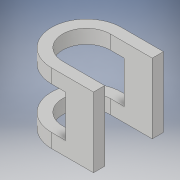
# Autodesk Inventor part: 410571040示範三
Saved by Autodesk Inventor 2017 (Build 210142000, 142)
## iProperties
Part Number: 410571040示範三
Material: 一般
Document SubType Name: Modeling
Designer: user
Density: 1 g/cm^3
Appearance: 預設
Author: user
Autodesk Inventor part; units mm, degrees
ref_plane "YZ Plane" through (0, 0, 0) normal (1, 0, 0) x (0, 1, 0)
ref_plane "XZ Plane" through (0, 0, 0) normal (0, 1, 0) x (-1, 0, 0)
ref_plane "XY Plane" through (0, 0, 0) normal (0, 0, 1) x (1, 0, 0)
sketch "草圖1" plane through (0, 0, 0) normal (0, 1, 0) x (-1, 0, 0)
  line L0 (0, 0) -> (-8, 0)
  line L1 (-8, 0) -> (-8, -30)
  line L2 (0, 0) -> (0, -30)
  arc A0 (-42, -30) -> (-8, -30) centre (-25, -30) ccw
  arc A1 (-50, -30) -> (0, -30) centre (-25, -30) ccw
  line L3 (6.1696, -30) -> (-69.0697, -30) construction
  line L4 (-25, -30) -> (-25, -20.8656)
  line L5 (-42, 0) -> (-42, -30)
  line L6 (-50, 0) -> (-50, -30)
  line L7 (-42, 0) -> (-50, 0)
  dimension "d8" = 30
  dimension "d9" = 8
  dimension "d10" = 25
  dimension "d11" = 17
  constraints: 16 end point, 4 point on circle, 4 point on line, 2 centre point, 2 horizontal, 2 perpendicular, 2 symmetric about line, 2 vertical, 1 coincident
  measures "d8" distance of L0.start L2.end
  measures "d9" distance of L0.start L0.end
  measures "d10" radius of A1
  measures "d11" radius of A0
extrude "擠出1" add sketch "草圖1" along normal blind 10
sketch "草圖2" plane through (0, 10, 0) normal (0, 1, 0) x (1, 0, 0)
  line L0 (0, 30) -> (0, 0) projected
  line L1 (0, 0) -> (0, 20)
  line L2 (0, 20) -> (8, 20)
  line L3 (8, 0) -> (8, 30) projected
  line L4 (8, 20) -> (8, 0)
  line L5 (8, 0) -> (0, 0)
  arc A0 (42, 30) -> (8, 30) centre (25, 30) ccw projected
  line L6 (25, 30) -> (25, 60.7006)
  line L7 (50, 20) -> (50, 0)
  line L8 (50, 0) -> (50, 20)
  line L9 (50, 20) -> (42, 20)
  line L10 (42, 0) -> (42, 20)
  line L11 (42, 20) -> (42, 0)
  line L12 (42, 0) -> (50, 0)
  point P0 (50, 30)
  dimension "d14" = 20
  constraints: 22 end point, 5 symmetric about line, 2 point on line, 2 vertical, 1 horizontal, 1 perpendicular
  measures "d14" distance of L12.start L10.end
extrude "擠出2" add sketch "草圖2" along normal blind 30
sketch "草圖3" plane through (0, 40, 0) normal (0, 1, 0) x (1, 0, 0)
  line L0 (0, 20) -> (8, 20) projected
  line L1 (8, 20) -> (8, 30) projected
  arc A0 (42, 30) -> (8, 30) centre (25, 30) ccw projected
  line L2 (42, 30) -> (42, 20) projected
  line L3 (42, 20) -> (50, 20) projected
  line L4 (50, 20) -> (50, 30) projected
  arc A1 (50, 30) -> (0, 30) centre (25, 30) ccw projected
  line L5 (0, 30) -> (0, 20) projected
  line L6 (0, 0) -> (8, 0) projected
  line L7 (8, 0) -> (8, 20) projected
  line L8 (8, 20) -> (0, 20) projected
  line L9 (0, 20) -> (0, 0) projected
  line L10 (50, 0) -> (50, 20) projected
  line L11 (50, 20) -> (42, 20) projected
  line L12 (42, 20) -> (42, 0) projected
  line L13 (42, 0) -> (50, 0) projected
extrude "擠出3" add sketch "草圖3" along normal blind 10
